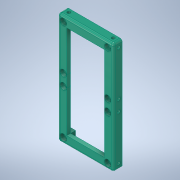
# Autodesk Inventor part: 10_Lid_el_2x1_v2
Saved by Autodesk Inventor 2022 (Build 260153000, 153)
## iProperties
Created: 2019-07-01
Part Number: 10_Lid_el_2x1_v2
Material: Generic
Document SubType Name: Modeling
Designer: diederichbenedict
Density: 1 g/cm^3
Appearance: IPHT_Türkis
Author: diederichbenedict
Autodesk Inventor part; units mm, degrees
ref_plane "YZ Plane" through (0, 0, 0) normal (1, 0, 0) x (0, 1, 0)
ref_plane "XZ Plane" through (0, 0, 0) normal (0, 1, 0) x (-1, 0, 0)
ref_plane "Work Plane1" through (0, 41.8, 0) normal (0, 0, 1) x (1, 0, 0)
sketch "Sketch1" plane through (0, 41.8, 0) normal (0, 0, 1) x (1, 0, 0)
  circle A0 centre (0.9, -0.9) radius 1.45 construction
  line L0 (4, -1.5) -> (1.5, -4) construction
  line L1 (4, -1.5) -> (4, 4) construction
  line L2 (4, 4) -> (-2, 4) construction
  arc A1 (-2, 4) -> (-4, 2) centre (-2, 2) ccw construction
  line L3 (-4, 2) -> (-4, -4) construction
  line L4 (-4, -4) -> (1.5, -4) construction
  arc A2 (45.8, 2) -> (43.8, 4) centre (43.8, 2) ccw construction
  line L5 (43.8, 4) -> (37.8, 4) construction
  line L6 (37.8, 4) -> (37.8, -1.5) construction
  line L7 (40.3, -4) -> (45.8, -4) construction
  line L8 (45.8, -4) -> (45.8, 2) construction
  circle A3 centre (40.9, -0.9) radius 1.45 construction
  line L9 (37.8, -40.3) -> (40.3, -37.8) construction
  line L10 (37.8, -40.3) -> (37.8, -45.8) construction
  line L11 (37.8, -45.8) -> (43.8, -45.8) construction
  arc A4 (43.8, -45.8) -> (45.8, -43.8) centre (43.8, -43.8) ccw construction
  line L12 (45.8, -43.8) -> (45.8, -37.8) construction
  line L13 (45.8, -37.8) -> (40.3, -37.8) construction
  circle A5 centre (40.9, -40.9) radius 1.45 construction
  circle A6 centre (0.9, -40.9) radius 1.45 construction
  line L14 (1.5, -37.8) -> (4, -40.3) construction
  line L15 (1.5, -37.8) -> (-4, -37.8) construction
  line L16 (-4, -37.8) -> (-4, -43.8) construction
  arc A7 (-4, -43.8) -> (-2, -45.8) centre (-2, -43.8) ccw construction
  line L17 (-2, -45.8) -> (4, -45.8) construction
  line L18 (4, -45.8) -> (4, -40.3) construction
  line L19 (40.3, -4) -> (37.8, -1.5) construction
  line L20 (-2, 54) -> (43.8, 54)
  line L21 (45.8, 52) -> (45.8, -43.8)
  line L22 (43.8, -45.8) -> (-2, -45.8)
  line L23 (-4, -43.8) -> (-4, 52)
  line L24 (40.3, -37.8) -> (40.3, 46)
  line L25 (37.8, 48.5) -> (4, 48.5)
  line L26 (1.5, 46) -> (1.5, -37.8)
  line L27 (4, -40.3) -> (37.8, -40.3)
  line L28 (37.8, -40.3) -> (40.3, -37.8)
  line L29 (4, -40.3) -> (1.5, -37.8)
  line L30 (4, 48.5) -> (1.5, 46)
  line L31 (40.3, 46) -> (37.8, 48.5)
  arc A8 (45.8, 52) -> (43.8, 54) centre (43.8, 52) ccw
  arc A9 (43.8, -45.8) -> (45.8, -43.8) centre (43.8, -43.8) ccw
  arc A10 (-4, -43.8) -> (-2, -45.8) centre (-2, -43.8) ccw
  arc A11 (-2, 54) -> (-4, 52) centre (-2, 52) ccw
  circle A12 centre (1, -1) radius 1.4
  circle A13 centre (40.8, -1) radius 1.4
  circle A14 centre (40.8, -40.8) radius 1.4
  circle A15 centre (1, -40.8) radius 1.4
  circle A16 centre (20.9, 29.1) radius 19.4 construction
  line L32 (4, 46) -> (4, -37.8)
  line L33 (4, -37.8) -> (37.8, -37.8)
  line L34 (37.8, -37.8) -> (37.8, 46)
  line L35 (37.8, 46) -> (4, 46)
  point P0 (45.8, -45.8)
  point P1 (45.8, 54)
  point P2 (-4, -45.8)
  point P3 (40.3, -40.3)
  point P4 (40.3, 48.5)
  point P5 (1.5, 48.5)
  point P6 (1.5, -40.3)
  point P7 (40.8, 49)
  dimension "d34" = 49.8
  dimension "d35" = 99.8
  dimension "d36" = 5.5
  dimension "d37" = 2.5
  dimension "d38" = 2.5
  dimension "d39" = 2.5
  dimension "d40" = 2.5
  dimension "d41" = 2.5
  dimension "d42" = 2.5
  dimension "d43" = 2.5
  dimension "d44" = 2.5
  dimension "d45" = 2
  dimension "d46" = 5
  dimension "d47" = 5
  dimension "d48" = 5
  dimension "d49" = 5
  dimension "d50" = 5
  dimension "d51" = 5
  dimension "d52" = 0.5
  dimension "d53" = 5
  dimension "d54" = 5
  dimension "d55" = 2.8
  dimension "d56" = 2.8
  dimension "d57" = 2.8
  dimension "d58" = 2.8
  dimension "d90" = 8
  constraints: 32 end point, 14 point on line, 11 tangent, 9 centre point, 8 point on circle, 6 parallel, 3 coincident, 3 equal radius, 3 perpendicular, 1 horizontal, 6 other
  measures "d34" distance of point (45.8, -45.8) point (-4, -45.8)
  measures "d35" distance of point (45.8, 54) point (45.8, -45.8)
  measures "d36" distance between parallel lines of L21 L24
  measures "d37" distance of L27.end point (40.3, -40.3)
  measures "d38" distance of L24.start point (40.3, -40.3)
  measures "d39" distance of L27.start point (1.5, -40.3)
  measures "d40" distance of L26.end point (1.5, -40.3)
  measures "d41" distance of L25.end point (1.5, 48.5)
  measures "d42" distance of L26.start point (1.5, 48.5)
  measures "d43" distance of L24.end point (40.3, 48.5)
  measures "d44" distance of L25.start point (40.3, 48.5)
  measures "d45" radius of A8
  measures "d46" distance from line of point (1, -40.8) L23
  measures "d47" distance from line of L22 point (1, -40.8)
  measures "d48" distance from line of L21 point (40.8, -40.8)
  measures "d49" distance from line of L22 point (40.8, -40.8)
  measures "d50" distance from line of L8 point (40.8, 49)
  measures "d51" distance from line of L20 point (40.8, 49)
  measures "d52" distance from line of point (1, -1) L26
  measures "d53" distance from line of L3 point (1, -1)
  measures "d54" distance from line of L2 point (1, -1)
  measures "d55" diameter of A12
  measures "d56" diameter of A13
  measures "d57" diameter of A14
  measures "d58" diameter of A15
  measures "d90" distance between parallel lines of L23 L32
extrude "Extrusion1" add sketch "Sketch1" along normal blind 8 contours L20 A8 L21 A9 L22 A10 L23 A11 | L28 L27 L29 L26 A12 L30 L25 L31 L24 A13
fillet "Fillet1" radius 2 8 edges at (20.9, -4, 8) (45.2142, -3.4142, 8) (45.8, 45.9, 8) (45.2142, 95.2142, 8) (20.9, 95.8, 8) (-3.4142, 95.2142, 8) (-4, 45.9, 8) (-3.4142, -3.4142, 8)
sketch "Sketch2" plane through (-2, -4, 0) normal (0, -1, 0) x (1, 0, 0)
  line L0 (43.8, -4.8712) -> (42.35, -4)
  line L1 (2, -4.8712) -> (0.55, -4)
  line L2 (-2, 0) -> (-2, 6) construction
  line L3 (45.8, 8) -> (0, 8) construction
  line L4 (47.8, 0) -> (47.8, 6) construction
  point P0 (2, 0)
  point P1 (3, 3.1)
  point P2 (42.8, 3.1)
  dimension "d59" = 5
  dimension "d60" = 4.9
  dimension "d61" = 5
  dimension "d62" = 4.9
  constraints: 4 end point, 6 other
  measures "d59" distance from line of point (3, 3.1) L2
  measures "d60" distance from line of point (3, 3.1) L3
  measures "d61" distance from line of point (42.8, 3.1) L4
  measures "d62" distance from line of point (42.8, 3.1) L3
hole "Hole1" at (40.8, -4, 3.1) at (1, -4, 3.1) direction (0, 1, 0) diameter 2.9 depth 6.5 tip angle 118
sketch "Sketch3" plane through (0, 41.8, 8) normal (0, 0, 1) x (1, 0, 0)
  circle A0 centre (20.9, -20.9) radius 16.9 construction
  point P0 (0, -41.8)
  constraints: 1 centre point
sketch "Sketch4" plane through (0, 41.8, 8) normal (0, 0, 1) x (1, 0, 0)
  circle A0 centre (1, -40.8) radius 1.4 projected
  circle A1 centre (40.8, -40.8) radius 1.4 projected
  circle A2 centre (40.8, -1) radius 1.4 projected
  circle A3 centre (1, -1) radius 1.4 projected
  circle A4 centre (1, -1) radius 1.4 construction
  circle A5 centre (40.8, -1) radius 1.4 construction
  circle A6 centre (40.8, -40.8) radius 1.4 construction
  circle A7 centre (1, -40.8) radius 1.4 construction
  line L0 (4, 46) -> (37.8, 46) construction
  line L1 (37.8, 46) -> (37.8, -37.8) construction
  line L2 (37.8, -37.8) -> (4, -37.8) construction
  line L3 (4, -37.8) -> (4, 46) construction
  line L4 (43.8, -43.8) -> (-2, -43.8) construction
  line L5 (43.8, 52) -> (43.8, -43.8) construction
  line L6 (-2, 52) -> (43.8, 52) construction
  line L7 (-2, -43.8) -> (-2, 52) construction
  line L8 (-4, 52) -> (-4, -43.8) construction
  line L9 (-4, 4.1) -> (45.187, 4.1) construction
  line L10 (-2, -45.8) -> (43.8, -45.8) construction
  circle A8 centre (1, 49) radius 1.4
  circle A9 centre (40.8, 49) radius 1.4
  circle A10 centre (40.8, 9.2) radius 1.4
  circle A11 centre (1, 9.2) radius 1.4
  circle A12 centre (1, 9.2) radius 1.4 construction
  circle A13 centre (40.8, 9.2) radius 1.4 construction
  circle A14 centre (40.8, 49) radius 1.4 construction
  circle A15 centre (1, 49) radius 1.4 construction
  line L11 (37.8, 46) -> (4, 46) construction
  line L12 (43.8, 52) -> (-2, 52) construction
  line L13 (-2, 54) -> (43.8, 54) construction
  line L14 (45.8, -43.8) -> (45.8, 52) projected
  dimension "d95" = 49.9
  dimension "d102" = 5
  dimension "d103" = 5
  dimension "d104" = 39.8
  dimension "d105" = 39.8
  dimension "d106" = 5
  dimension "d107" = 10.2
  constraints: 10 symmetric about line, 8 centre point, 8 end point, 1 horizontal, 1 midpoint, 8 other
  measures "d95" distance between parallel lines of L9 L10
  measures "d102" distance from line of A14.centre L13
  measures "d103" distance from line of A9.centre L14
  measures "d104" distance of A10.centre A14.centre
  measures "d105" distance of A2.centre A1.centre
  measures "d106" distance from line of A1.centre L10
  measures "d107" distance of A2.centre A10.centre
hole "Hole2" at (1, 40.8, 8) at (1, 1, 8) at (40.8, 1, 8) at (40.8, 40.8, 8) at (1, 51, 8) at (1, 90.8, 8) at (40.8, 90.8, 8) at (40.8, 51, 8) direction (0, 0, -1) diameter 2.9 depth 12 tip angle 118 counterbore diameter 6 counterbore depth 3.1
chamfer "Chamfer2" distance 4.5 angle 45 2 edges at (4, 45.9, 0) (37.8, 45.9, 0)
sketch "Sketch6" plane through (-4, -2, 0) normal (-1, 0, 0) x (0, 0, 1)
  line L0 (0, -2) -> (6, -2) construction
  line L1 (8, 0) -> (8, 95.8) construction
  line L2 (0, 97.8) -> (6, 97.8) construction
  circle A0 centre (3.1, 92.8) radius 1.4 construction
  circle A1 centre (3.1, 3) radius 1.4 construction
  line L3 (4.5, 89.8) -> (4.5, 6) construction
  line L4 (3.1, 3) -> (3.1, 43) construction
  line L5 (3.1, 92.8) -> (3.1, 52.8) construction
  circle A2 centre (3.1, 43) radius 1.4 construction
  circle A3 centre (3.1, 52.8) radius 1.4 construction
  point P0 (0, 2)
  dimension "d63" = 2.8
  dimension "d64" = 2.8
  dimension "d65" = 4.9
  dimension "d66" = 5
  dimension "d67" = 5
  dimension "d68" = 4.9
  dimension "d97" = 40
  dimension "d98" = 40
  constraints: 4 centre point, 4 end point, 2 coincident, 2 parallel, 2 tangent
  measures "d63" diameter of A0
  measures "d64" diameter of A1
  measures "d65" distance from line of L5.start L1
  measures "d66" distance from line of L5.start L2
  measures "d67" distance from line of L4.start L0
  measures "d68" distance from line of L1 L4.start
  measures "d97" distance of L4.start L4.end
  measures "d98" distance of L5.start L5.end
hole "Hole3" at (-4, 90.8, 3.1) at (-4, 1, 3.1) at (-4, 41, 3.1) at (-4, 50.8, 3.1) direction (1, 0, 0) diameter 2.8 depth 6.5 tip angle 118
sketch "Sketch7" plane through (45.8, -2, 0) normal (1, 0, 0) x (0, 0, -1)
  circle A0 centre (-3.1, 92.8) radius 1.4 projected
  circle A1 centre (-3.1, 3) radius 1.4 projected
  circle A2 centre (-3.1, 43) radius 1.4 projected
  circle A3 centre (-3.1, 52.8) radius 1.4 projected
  point P0 (0, 2)
  constraints: 1 vertical alignment
hole "Hole4" at (45.8, 90.8, 3.1) at (45.8, 1, 3.1) at (45.8, 41, 3.1) at (45.8, 50.8, 3.1) direction (-1, 0, 0) diameter 2.8 depth 6.5 tip angle 118
sketch "Sketch8" plane through (-2, 95.8, 0) normal (0, 1, 0) x (1, 0, 0)
  circle A0 centre (3, -3.1) radius 1.45 projected
  circle A1 centre (42.8, -3.1) radius 1.45 projected
  point P0 (2, 0)
  point P1 (4.45, -3.1)
  point P2 (4.45, -3.1)
  point P3 (44.25, -3.1)
  point P4 (44.25, -3.1)
hole "Hole5" at (1, 95.8, 3.1) at (40.8, 95.8, 3.1) direction (0, -1, 0) diameter 2.8 depth 6.5 tip angle 118
sketch "Sketch9" plane through (37.8, 4, 8) normal (-1, 0, 0) x (0, 0, 1)
  line L0 (-8, 0) -> (-3.5, 0) projected
  line L1 (-3.5, 83.8) -> (-8, 83.8) projected
  line L2 (-3.5, 0) -> (-8, -4.5)
  line L3 (-8, 89.8) -> (-8, -6) projected
  line L4 (-3.5, 0) -> (2.864, 0) construction
  line L5 (-8, -4.5) -> (-8, 0)
  line L6 (-3.5, 83.8) -> (-8, 88.3)
  line L7 (-3.5, 83.8) -> (2.864, 83.8) construction
  line L8 (-8, 88.3) -> (-8, 83.8)
  line L9 (-8, 83.8) -> (-3.5, 83.8)
  point P0 (-8, -4)
  dimension "d91" = 135
  dimension "d92" = 135
  constraints: 14 end point, 3 collinear, 2 equal length, 2 horizontal, 2 point on line
  measures "d91" angle of L2 L4
  measures "d92" angle of L7 L6
extrude "Extrusion3" cut sketch "Sketch9" along normal up to surface (33.8 mm away)
equation "\"d38\" = d37"
equation "\"d39\" = d37"
equation "\"d40\" = d39"
equation "\"d41\" = d37"
equation "\"d42\" = d41"
equation "\"d43\" = d37"
equation "\"d44\" = d43"
body "Solid1"
